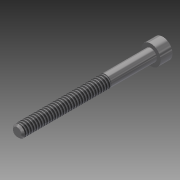
# Autodesk Inventor part: 6-32 SHCS x1750 - .205
Saved by Autodesk Inventor 2015 (Build 190159000, 159)
## iProperties
Created: 2012-09-29
Part Number: 6-32 SHCS x1750 - .205
Material: Stainless Steel
Document SubType Name: Modeling
Designer: Nemo
Density: 1 g/cm^3
Appearance: Semi-Polished
Author: Nemo
Autodesk Inventor part; units mm, degrees
ref_plane "YZ Plane" through (0, 0, 0) normal (1, 0, 0) x (0, 1, 0)
ref_plane "XZ Plane" through (0, 0, 0) normal (0, 1, 0) x (-1, 0, 0)
ref_plane "XY Plane" through (0, 0, 0) normal (0, 0, 1) x (1, 0, 0)
sketch "Sketch1" plane through (0, 0, 0) normal (0, 0, 1) x (1, 0, 0)
  circle A0 centre (0, 0) radius 1.7526
  dimension "d0" = 3.5052
  constraints: 1 centre point, 1 coincident
  measures "d0" diameter of A0
extrude "Extrusion1" add sketch "Sketch1" along normal blind 39.243
sketch "Sketch2" plane through (0, 0, 0) normal (0, 0, -1) x (-1, 0, 0)
  circle A0 centre (0, 0) radius 1.7526 construction
  circle A1 centre (0, 0) radius 2.8702
  dimension "d3" = 5.7404
  constraints: 1 centre point, 1 coincident
  measures "d3" diameter of A1
extrude "Extrusion2" add sketch "Sketch2" along normal blind 3.5052
sketch "Sketch3" plane through (0, 0, -3.5052) normal (0, 0, -1) x (-1, 0, 0)
  circle A0 centre (0, 0) radius 2.8702 projected
  line L0 (0, 1.604) -> (1.3891, 0.802)
  line L1 (1.3891, 0.802) -> (1.3891, -0.802)
  line L2 (1.3891, -0.802) -> (0, -1.604)
  line L3 (0, -1.604) -> (-1.3891, -0.802)
  line L4 (-1.3891, -0.802) -> (-1.3891, 0.802)
  line L5 (-1.3891, 0.802) -> (0, 1.604)
  dimension "d6" = 2.7781
  constraints: 12 end point, 1 coincident, 13 other
  measures "d6" distance between parallel lines of L1 L4
extrude "Extrusion3" cut sketch "Sketch3" against normal blind 1.7526 contours L0 L1 L2 L3 L4 L5
chamfer "Chamfer1" distance 0.508 angle 45 1 edges at (-1.7526, 0, 39.243)
thread "Thread2" size "6-32 UNC" class "2A" standard "ANSI Unified Screw Threads" length 25.4
body "Solid1"
